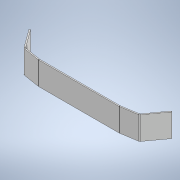
# Autodesk Inventor part: FRONT
Saved by Autodesk Inventor 2020 (Build 240168000, 168)
## iProperties
Created: 2022-07-14
Part Number: FRONT
Material: Generic
Document SubType Name: Sheet Metal
Designer: karimi2
Density: 1 g/cm^3
Sheet Metal Rule: Default_mm
Appearance: Default
Author: karimi2
Autodesk Inventor part; units mm, degrees
ref_plane "YZ Plane" through (0, 0, 0) normal (1, 0, 0) x (0, 1, 0)
ref_plane "XZ Plane" through (0, 0, 0) normal (0, 1, 0) x (-1, 0, 0)
ref_plane "XY Plane" through (0, 0, 0) normal (0, 0, 1) x (1, 0, 0)
sketch "Sketch1" plane through (0, 0, 0) normal (0, 0, 1) x (1, 0, 0)
  line L0 (0, 0) -> (-140, 0)
  line L1 (-140, 0) -> (-140, 40)
  line L2 (-140, 40) -> (0, 40)
  line L3 (0, 40) -> (0, 0) construction
  line L4 (0, 0) -> (140, 0)
  line L5 (140, 0) -> (140, 40)
  line L6 (140, 40) -> (0, 40)
  dimension "d0" = 140
  dimension "d1" = 40
  measures "d0" distance of L1.end L2.end
  measures "d1" distance of L0.end L1.end
extrude "Plate1" add sketch "Sketch1" along normal blind 2
sketch "Sketch2" plane through (0, 0, 2) normal (0, 0, 1) x (1, 0, 0)
  line L0 (-100, 40) -> (-100, 0)
  line L1 (100, 40) -> (100, 0)
  point P0 (0, 0)
  dimension "d3" = 40
  dimension "d4" = 100
  dimension "d5" = 100
  dimension "d6" = 40
  constraints: 4 end point, 2 vertical
  measures "d3" distance of L0.start L0.end
  measures "d4" distance from line of point (0, 0) L0
  measures "d5" distance from line of point (0, 0) L1
  measures "d6" distance of L1.start L1.end
fold "Fold1" angle 45 bend radius 2 thickness 2 k factor 0.44 line from (-100, 40, 2) to (-100, 0, 2) line at bend centre moving side (-1, 0, 0) folds toward (0, 0, -1)
fold "Fold2" angle 45 bend radius 2 thickness 2 k factor 0.44 line from (100, 40, 2) to (100, 0, 2) line at bend centre moving side (1, 0, 0) folds toward (0, 0, -1)
sketch "Sketch3" plane through (0, 0, 2) normal (0, 0, 1) x (1, 0, 0)
  line L0 (-98.869, 40) -> (98.869, 40) projected
  line L1 (70, 40) -> (70, 0)
  line L2 (-70, 40) -> (-70, 0)
  point P0 (0, 0)
  dimension "d19" = 70
  dimension "d20" = 40
  dimension "d21" = 70
  dimension "d22" = 40
  constraints: 4 end point, 2 point on line, 2 vertical
  measures "d19" distance from line of point (0, 0) L2
  measures "d20" distance of L2.start L2.end
  measures "d21" distance from line of point (0, 0) L1
  measures "d22" distance of L1.start L1.end
fold "Fold3" angle 9 bend radius 2 thickness 2 k factor 0.44 line from (70, 40, 2) to (70, 0, 2) line at bend centre moving side (1, 0, 0) folds toward (0, 0, -1)
fold "Fold4" angle 9 bend radius 2 thickness 2 k factor 0.44 line from (-70, 40, 2) to (-70, 0, 2) line at bend centre moving side (-1, 0, 0) folds toward (0, 0, -1)
equation "\"d2\" = Thickness"
equation "\"d7\" = BendReliefWidth"
equation "\"d8\" = BendReliefDepth"
equation "\"d9\" = MinimumRemnant"
equation "\"d10\" = TransitionRadius"
equation "\"d12\" = BendRadius"
equation "\"d13\" = BendReliefWidth"
equation "\"d14\" = BendReliefDepth"
equation "\"d15\" = MinimumRemnant"
equation "\"d16\" = TransitionRadius"
equation "\"d18\" = BendRadius"
equation "\"d23\" = BendReliefWidth"
equation "\"d24\" = BendReliefDepth"
equation "\"d25\" = MinimumRemnant"
equation "\"d26\" = TransitionRadius"
equation "\"d28\" = BendRadius"
equation "\"d29\" = BendReliefWidth"
equation "\"d30\" = BendReliefDepth"
equation "\"d31\" = MinimumRemnant"
equation "\"d32\" = TransitionRadius"
equation "\"d34\" = BendRadius"
equation "\"BendRadius\" = Thickness"
equation "\"BendReliefWidth\" = Thickness"
equation "\"BendReliefDepth\" = 0.5 * Thickness"
equation "\"CornerReliefSize\" = 4 * Thickness"
equation "\"MinimumRemnant\" = 2 * Thickness"
equation "\"TransitionRadius\" = BendRadius"
equation "\"JacobiRadiusSize\" = BendRadius"
equation "\"GapSize\" = Thickness"
equation "\"Thickness\" = 2"
body "Solid1"
